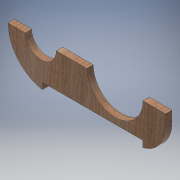
# Autodesk Inventor part: cannon support front
Saved by Autodesk Inventor 2018 (Build 220112000, 112)
## iProperties
Created: 2017-05-03
Part Number: cannon support front
Material: Generic
Document SubType Name: Modeling
Designer: gsegs
Density: 1 g/cm^3
Appearance: Birch - Natural Polished
Author: gsegs
Autodesk Inventor part; units mm, degrees
ref_plane "YZ Plane" through (0, 0, 0) normal (1, 0, 0) x (0, 1, 0)
ref_plane "XZ Plane" through (0, 0, 0) normal (0, 1, 0) x (-1, 0, 0)
ref_plane "XY Plane" through (0, 0, 0) normal (0, 0, 1) x (1, 0, 0)
sketch "Sketch1" plane through (0, 0, 0) normal (0, 0, 1) x (1, 0, 0)
  line L0 (0, 101.6) -> (50.8, 101.6)
  line L1 (466.725, 101.6) -> (466.725, 66.675)
  line L2 (466.725, 0) -> (400.05, 0) construction
  line L3 (0, 0) -> (0, 101.6) construction
  arc A0 (50.8, 101.6) -> (142.875, 101.6) centre (96.8375, 101.6) ccw
  arc A1 (233.3625, 101.6) -> (400.05, 101.6) centre (316.7062, 101.6) ccw
  line L4 (50.8, 101.6) -> (142.875, 101.6) construction
  line L5 (142.875, 101.6) -> (233.3625, 101.6)
  line L6 (233.3625, 101.6) -> (400.05, 101.6) construction
  line L7 (400.05, 101.6) -> (466.725, 101.6)
  arc A2 (0, 101.6) -> (101.6, 0) centre (101.6, 101.6) ccw
  arc A3 (400.05, 0) -> (466.725, 66.675) centre (400.05, 66.675) ccw
  line L8 (400.05, 0) -> (101.6, 0)
  line L9 (466.725, 66.675) -> (466.725, 0) construction
  line L10 (101.6, 0) -> (0, 0) construction
  dimension "d0" = 466.725
  dimension "d1" = 101.6
  dimension "d2" = 50.8
  dimension "d3" = 90.4875
  dimension "d4" = 66.675
  dimension "d5" = 92.075
  dimension "d6" = 166.6875
  constraints: 22 end point, 17 parallel, 11 point on line, 10 perpendicular, 8 point on circle, 8 tangent, 5 horizontal, 4 centre point, 2 midpoint, 1 coincident, 1 line through centre, 1 vertical alignment
  measures "d0" distance between parallel lines of L1 L3
  measures "d1" distance between parallel lines of L2 L0
  measures "d2" distance of L0.end L0.start
  measures "d3" distance of L5.end L4.end
  measures "d4" distance of L1.start L6.end
  measures "d5" distance of L4.end L0.end
  measures "d6" distance of L6.end L5.end
extrude "Extrusion1" add sketch "Sketch1" along normal blind 19.05
sketch "Sketch2" plane through (0, 0, 19.05) normal (0, 0, 1) x (1, 0, 0)
  line L0 (101.6, 0) -> (101.6, -19.05) projected
  arc A0 (0, 101.6) -> (101.6, 0) centre (101.6, 101.6) ccw projected
  line L1 (400.05, 0) -> (400.05, -19.05) projected
  arc A1 (400.05, 0) -> (466.725, 66.675) centre (400.05, 66.675) ccw projected
  arc A2 (400.05, -19.05) -> (466.725, 66.675) centre (378.2786, 66.675) ccw
  line L2 (466.725, 66.675) -> (466.725, 101.6) projected
  arc A3 (0, 101.6) -> (101.6, -19.05) centre (122.4359, 101.6) ccw
  line L3 (0, 101.6) -> (0, 165.1)
  point P0 (0, 0)
  constraints: 4 point on circle, 3 tangent, 2 centre point, 2 end point, 1 vertical
extrude "Extrusion2" add sketch "Sketch2" against normal up to surface (19.05 mm away)
body "Solid1"
